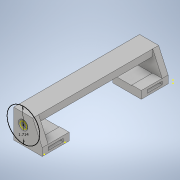
# Autodesk Inventor part: GRAVVY FRONT
Saved by Autodesk Inventor 2020 (Build 240168000, 168)
## iProperties
Created: 2019-11-03
Part Number: GRAVVY FRONT
Material: Generic
Document SubType Name: Modeling
Designer: Arman Ahmad
Density: 1 g/cm^3
Appearance: Default
Author: Arman Ahmad
## iProperties of the stored document _3DPrint.ipt
Created: 2020-02-16
Part Number: _3DPrint
Material: Generic
Document SubType Name: Modeling
Designer: akend
Density: 1 g/cm^3
Appearance: Default
Author: akend
Autodesk Inventor part; units mm, degrees
ref_plane "YZ Plane" through (0, 0, 0) normal (1, 0, 0) x (0, 1, 0)
ref_plane "XZ Plane" through (0, 0, 0) normal (0, 1, 0) x (-1, 0, 0)
ref_plane "XY Plane" through (0, 0, 0) normal (0, 0, 1) x (1, 0, 0)
sketch "Sketch1" plane through (0, 0, 0) normal (0, 1, 0) x (-1, 0, 0)
  line L0 (41.275, -164.3062) -> (9.525, -164.3062)
  line L1 (9.525, -164.3062) -> (9.525, -11.9062)
  line L2 (9.525, -11.9062) -> (41.275, -11.9062)
  line L3 (41.275, -11.9062) -> (41.275, -164.3062)
  line L4 (41.275, -164.3062) -> (9.525, -164.3062)
  line L5 (9.525, -164.3062) -> (9.525, -146.7428)
  line L6 (9.525, -146.7428) -> (41.275, -146.7428)
  line L7 (41.275, -146.7428) -> (41.275, -164.3062)
  point P0 (0, 0)
  dimension "d37" = 31.75
  dimension "d50" = 152.4
  constraints: 16 end point, 4 parallel, 2 horizontal, 2 perpendicular, 1 point on line
  measures "d37" distance between parallel lines of L1 L3
  measures "d50" distance between parallel lines of L0 L2
sketch "Sketch2" plane through (0, 0, 0) normal (1, 0, 0) x (0, 1, 0)
  point P0 (0, 0)
extrude "Extrusion1" add sketch "Sketch1" along normal mid plane 7.62
sketch "Sketch3" plane through (0, 3.81, 0) normal (0, 1, 0) x (1, 0, 0)
  point P0 (0, 0)
sketch "Sketch4" plane through (0, 3.81, 0) normal (0, 1, 0) x (1, 0, 0)
  line L0 (-47.625, 3.9687) -> (-47.625, 172.2437)
  line L1 (-47.625, 172.2437) -> (-3.175, 172.2437)
  line L2 (-3.175, 172.2437) -> (-3.175, 3.9688)
  line L3 (-41.275, 164.3062) -> (-9.525, 164.3062) projected
  line L4 (-41.275, 11.9062) -> (-41.275, 164.3062) projected
  line L5 (-9.525, 164.3062) -> (-41.275, 164.3062) projected
  line L6 (-41.275, 11.9062) -> (-9.525, 11.9062) projected
  line L7 (-41.275, 164.3062) -> (-9.525, 164.3062)
  line L8 (-9.525, 164.3062) -> (-9.525, 11.9062)
  line L9 (-9.525, 11.9062) -> (-41.275, 11.9062)
  line L10 (-41.275, 11.9062) -> (-41.275, 164.3062)
  line L11 (-47.625, 3.9687) -> (-3.175, 3.9688)
  dimension "d38" = 7.9375
  dimension "d40" = 7.9375
  dimension "d41" = 6.35
  dimension "d42" = 6.35
  constraints: 16 end point, 4 parallel, 1 horizontal, 1 perpendicular, 1 vertical
  measures "d38" distance between parallel lines of L3 L1
  measures "d40" distance between parallel lines of L11 L6
  measures "d41" distance between parallel lines of L4 L0
  measures "d42" distance between parallel lines of L8 L2
extrude "Extrusion2" add sketch "Sketch4" against normal blind 38.1
fillet "Fillet1" radius 3.175 3 edges at (-47.625, -34.29, -88.1062) (-47.625, -15.24, -3.9687) (-47.625, -15.24, -172.2437)
sketch "Sketch6" plane through (-3.175, 3.81, -3.9688) normal (1, 0, 0) x (0, 0, -1)
  line L0 (140.3375, -7.0861) -> (160.3375, -7.0861)
  line L1 (160.3375, -7.0861) -> (160.3375, -3.0861)
  line L2 (160.3375, -3.0861) -> (140.3375, -3.0861)
  line L3 (140.3375, -3.0861) -> (140.3375, -7.0861)
  line L4 (27.3343, -7.0861) -> (7.3343, -7.0861)
  line L5 (7.3343, -7.0861) -> (7.3343, -3.0861)
  line L6 (7.3343, -3.0861) -> (27.3343, -3.0861)
  line L7 (27.3343, -3.0861) -> (27.3343, -7.0861)
  line L8 (85.181, -7.0861) -> (65.181, -7.0861)
  line L9 (65.181, -7.0861) -> (65.181, -3.0861)
  line L10 (65.181, -3.0861) -> (85.181, -3.0861)
  line L11 (85.181, -3.0861) -> (85.181, -7.0861)
  line L12 (0, 0) -> (168.275, 0) projected
  point P0 (-3.9688, -3.81)
  point P1 (160.3375, -38.1)
  dimension "d20" = 4
  dimension "d21" = 20
  dimension "d22" = 0
  dimension "d23" = 3.0861
  dimension "d24" = 3.0861
  constraints: 24 end point, 6 parallel, 3 equal length, 3 horizontal, 3 perpendicular, 2 point on line
  measures "d20" distance between parallel lines of L2 L0
  measures "d21" distance between parallel lines of L3 L1
  measures "d22" distance from line of point (160.337, -38.1) L1
  measures "d23" distance between parallel lines of L12 L2
  measures "d24" distance between parallel lines of L12 L10
extrude "Extrusion3" cut sketch "Sketch6" against normal blind 31.75 contours L3 L2 L1 L0
sketch "Sketch7" plane through (-3.175, 3.81, -3.9688) normal (1, 0, 0) x (0, 0, -1)
  line L0 (27.9375, -7.0861) -> (7.9375, -7.0861)
  line L1 (7.9375, -7.0861) -> (7.9375, -3.0861)
  line L2 (7.9375, -3.0861) -> (27.9375, -3.0861)
  line L3 (27.9375, -3.0861) -> (27.9375, -7.0861)
  line L4 (160.3375, -7.0861) -> (140.3375, -7.0861) projected
  line L5 (140.3375, -7.0861) -> (140.3375, -3.0861) projected
  line L6 (0, 0) -> (168.275, 0) projected
  line L7 (140.3375, -3.0861) -> (160.3375, -3.0861) projected
  point P0 (-3.9688, -3.81)
  point P1 (7.9375, -38.1)
  dimension "d28" = 0
  dimension "d31" = 3.0861
  constraints: 8 end point, 3 parallel, 2 equal length, 1 horizontal, 1 perpendicular
  measures "d28" distance from line of L1 point (7.937, -38.1)
  measures "d31" distance between parallel lines of L6 L2
extrude "Extrusion4" cut sketch "Sketch7" against normal blind 31.75
sketch "Sketch8" plane through (-3.175, 3.81, -3.9688) normal (1, 0, 0) x (0, 0, -1)
  line L0 (94.1324, -7.0861) -> (74.1324, -7.0861)
  line L1 (74.1324, -7.0861) -> (74.1324, -3.0861)
  line L2 (74.1324, -3.0861) -> (94.1324, -3.0861)
  line L3 (94.1324, -3.0861) -> (94.1324, -7.0861)
  line L4 (140.3375, -7.0861) -> (140.3375, -3.0861) projected
  line L5 (140.3375, -3.0861) -> (160.3375, -3.0861) projected
  line L6 (0, 0) -> (168.275, 0) projected
  line L7 (168.275, 0) -> (168.275, -38.1) projected
  line L8 (0, 0) -> (0, -38.1) projected
  point P0 (-3.9688, -3.81)
  point P1 (0, -38.1)
  dimension "d32" = 3.0861
  dimension "d33" = 74.1426
  constraints: 8 end point, 4 parallel, 1 horizontal, 1 perpendicular, 1 other
  measures "d32" distance between parallel lines of L6 L2
  measures "d33" distance between parallel lines of L7 L3
extrude "Extrusion5" cut sketch "Sketch8" against normal blind 31.75
sketch "Sketch10" plane through (-3.175, -34.29, -172.2437) normal (0, 0, -1) x (-1, 0, 0)
  point P0 (-3.175, 34.29)
  point P1 (24.9089, 14.3132)
hole "Hole3" at (-28.0839, -19.9768, -172.2437) direction (0, 0, 1) diameter 8.89 end through all
sketch "Sketch11" plane through (-3.175, -34.29, -172.2437) normal (0, 0, -1) x (-1, 0, 0)
  circle A0 centre (24.9089, 14.3132) radius 4.445 projected
  point P0 (-3.175, 34.29)
  constraints: 1 coincident
hole "Hole4" at (-28.0839, -19.9768, -172.2437) direction (0, 0, 1) diameter 12.7 depth 4.7625 tip angle 118
sketch "Sketch12" plane through (-3.175, -34.29, -3.9688) normal (0, 0, 1) x (1, 0, 0)
  point P0 (3.175, 34.29)
  point P1 (-25.0763, 13.995)
hole "Hole5" at (-28.2513, -20.295, -3.9688) direction (0, 0, -1) diameter 12.7 depth 4.7625 tip angle 118
sketch "Sketch13" plane through (-47.625, 3.81, -169.0687) normal (-1, 0, 0) x (0, 0, 1)
  line L0 (74.93, -14.0718) -> (86.995, -14.0718)
  line L1 (86.995, -14.0718) -> (86.995, -8.3898)
  line L2 (86.995, -8.3898) -> (74.93, -8.3898)
  line L3 (74.93, -8.3898) -> (74.93, -14.0718)
  line L4 (161.925, 0) -> (161.925, -34.925) projected
  line L5 (0, -34.925) -> (0, 0) projected
  point P0 (169.0687, -3.81)
  dimension "d72" = 74.93
  dimension "d73" = 74.93
  constraints: 8 end point, 2 parallel, 1 horizontal, 1 perpendicular
  measures "d72" distance between parallel lines of L4 L1
  measures "d73" distance between parallel lines of L5 L3
extrude "Extrusion6" add sketch "Sketch13" along normal blind 12.7
fillet "Fillet2" radius 1.27 1 edges at (-60.325, -10.2618, -88.1062)
fillet "Fillet3" radius 1.27 9 edges at (-60.325, -4.5798, -88.1062) (-59.953, -9.8898, -94.1387) (-60.325, -6.7858, -94.1387) (-53.34, -10.2618, -94.1387) (-53.975, -4.5798, -94.1387) (-59.953, -9.8898, -82.0737) (-60.325, -6.7858, -82.0737) (-53.34, -10.2618, -82.0737) (-53.975, -4.5798, -82.0737)
sketch "Sketch14" plane through (-47.625, -10.2618, -92.8687) normal (0, -1, 0) x (1, 0, 0)
  point P0 (47.625, 92.8687)
  point P1 (-5.4964, 5.0244)
hole "Hole6" at (-53.1214, -10.2618, -87.8444) direction (0, 1, 0) diameter 6.35 end through all
sketch "Sketch15" plane through (0, -34.29, 0) normal (0, -1, 0) x (1, 0, 0)
  line L0 (-3.175, -164.3062) -> (-34.925, -164.3062) projected
  line L1 (-3.175, -172.2437) -> (-3.175, -3.9688) projected
  line L2 (-9.6565, -164.3062) -> (-3.175, -164.3062)
  line L3 (-3.175, -164.3062) -> (-3.175, -12.0649)
  line L4 (-3.175, -12.0649) -> (-9.6565, -12.0649)
  line L5 (-9.6565, -12.0649) -> (-9.6565, -164.3062)
  point P0 (0, 0)
  constraints: 8 end point, 2 parallel, 2 point on line, 1 horizontal, 1 perpendicular
extrude "Extrusion7" cut sketch "Sketch15" against normal blind 21.59
sketch "Sketch16" plane through (0, -34.29, 0) normal (0, -1, 0) x (1, 0, 0)
  line L0 (-41.275, -11.9062) -> (-41.275, -164.3062) projected
  line L1 (-47.625, -169.0687) -> (-47.625, -7.1438) projected
  line L2 (-41.275, -164.3062) -> (-47.625, -164.3062)
  line L3 (-47.625, -164.3062) -> (-47.625, -11.6343)
  line L4 (-47.625, -11.6343) -> (-41.275, -11.6343)
  line L5 (-41.275, -11.6343) -> (-41.275, -164.3062)
  point P0 (0, 0)
  constraints: 8 end point, 2 parallel, 1 horizontal, 1 perpendicular, 1 point on line
extrude "Extrusion8" cut sketch "Sketch16" against normal blind 21.59
fillet "Fillet4" radius 1.27 4 edges at (-3.175, -34.29, -8.0168) (-3.175, -15.24, -3.9688) (-3.175, -34.29, -168.275) (-3.175, -15.24, -172.2437)
sketch "Sketch17" plane through (-44.45, -34.29, -3.9687) normal (0, 0, 1) x (1, 0, 0)
  line L0 (3.6661, -9.4735) -> (29.0661, -9.4735)
  line L1 (29.0661, -9.4735) -> (29.0661, 38.1)
  line L2 (29.0661, 38.1) -> (3.6661, 38.1)
  line L3 (3.6661, 38.1) -> (3.6661, -9.4735)
  circle A0 centre (16.3661, 14.3132) radius 4.445 projected
  line L4 (3.6661, -9.4735) -> (29.0661, 38.1) construction
  line L5 (29.0661, -9.4735) -> (3.6661, 38.1) construction
  line L6 (3.6661, 38.1) -> (-19.5186, 38.1)
  line L7 (-19.5186, 38.1) -> (-19.5186, -9.4735)
  line L8 (-19.5186, -9.4735) -> (3.6661, -9.4735)
  line L9 (3.6661, -9.4735) -> (3.6661, 38.1)
  line L10 (29.0661, 38.1) -> (55.1329, 38.1)
  line L11 (55.1329, 38.1) -> (55.1329, -9.4735)
  line L12 (55.1329, -9.4735) -> (29.0661, -9.4735)
  line L13 (29.0661, -9.4735) -> (29.0661, 38.1)
  point P0 (44.45, 34.29)
  point P1 (29.0661, -9.4735)
  point P2 (3.6661, -9.4735)
  dimension "d90" = 25.4
  constraints: 28 end point, 6 parallel, 3 horizontal, 3 perpendicular, 2 midpoint, 1 point on line
  measures "d90" distance of L0.start L0.end
extrude "Extrusion9" cut sketch "Sketch17" against normal blind 169.8625 contours L8 L7 L6 L3 | L1 L10 L11 L12
sketch "Sketch18" plane through (-15.3839, 3.81, -172.2437) normal (0, 0, -1) x (-1, 0, 0)
  circle A0 centre (12.7, -23.7868) radius 4.445 projected
  circle A1 centre (12.7, -23.7868) radius 21.7714
  point P0 (-15.3839, -3.81)
  dimension "d93" = 43.5429
  constraints: 1 centre point, 1 coincident
  measures "d93" diameter of A1
sketch "Sketch19" plane through (-34.925, -3.2761, -144.3062) normal (0, 0, -1) x (-1, 0, 0)
  point P0 (-34.925, 3.2761)
sketch "Sketch20" plane through (0, -3.81, 0) normal (0, -1, 0) x (1, 0, 0)
  line L0 (-40.7839, -164.3062) -> (-15.3839, -164.3062) projected
  line L1 (-40.7839, -11.9062) -> (-15.3839, -11.9062) projected
  line L2 (-40.7839, -164.3062) -> (-15.3839, -164.3062)
  line L3 (-15.3839, -164.3062) -> (-15.3839, -11.9062)
  line L4 (-15.3839, -11.9062) -> (-40.7839, -11.9062)
  line L5 (-40.7839, -11.9062) -> (-40.7839, -164.3062)
  point P0 (0, 0)
  constraints: 8 end point, 2 parallel, 1 horizontal, 1 perpendicular
extrude "Extrusion10" add sketch "Sketch20" along normal blind 3
sketch "Sketch21" plane through (0, -6.81, 0) normal (0, -1, 0) x (1, 0, 0)
  line L0 (-40.7839, -164.3062) -> (-40.7839, -172.2437) projected
  line L1 (-40.7839, -164.3062) -> (-34.4339, -164.3062)
  line L2 (-34.4339, -164.3062) -> (-34.4339, -11.9062)
  line L3 (-34.4339, -11.9062) -> (-40.7839, -11.9062)
  line L4 (-40.7839, -11.9062) -> (-40.7839, -164.3062)
  line L5 (-15.3839, -164.3062) -> (-21.7339, -164.3062)
  line L6 (-21.7339, -164.3062) -> (-21.7339, -11.9062)
  line L7 (-21.7339, -11.9062) -> (-15.3839, -11.9062)
  line L8 (-15.3839, -11.9062) -> (-15.3839, -164.3062)
  point P0 (0, 0)
  dimension "d96" = 6.35
  dimension "d97" = 6.35
  constraints: 16 end point, 4 parallel, 2 horizontal, 2 perpendicular, 1 point on line
  measures "d96" distance of L3.end L2.end
  measures "d97" distance of L6.end L7.end
extrude "Extrusion11" add sketch "Sketch21" along normal blind 8.255
sketch "Sketch22" plane through (-15.3839, -34.29, -3.9688) normal (1, 0, 0) x (0, 0, -1)
  point P0 (-3.9688, 34.29)
sketch "Sketch23" plane through (-15.3839, -34.29, -3.9688) normal (1, 0, 0) x (0, 0, -1)
  line L0 (168.275, 38.1) -> (0, 38.1) projected
  line L1 (0, 38.1) -> (35.8902, 38.1)
  line L2 (35.8902, 38.1) -> (35.8902, 27.9146)
  line L3 (35.8902, 27.9146) -> (0, 27.9146)
  line L4 (0, 27.9146) -> (0, 38.1)
  line L5 (168.275, 38.1) -> (132.3848, 38.1)
  line L6 (132.3848, 38.1) -> (132.3848, 27.9146)
  line L7 (132.3848, 27.9146) -> (168.275, 27.9146)
  line L8 (168.275, 27.9146) -> (168.275, 38.1)
  line L9 (7.9375, 35.0139) -> (7.9375, 31.0139) projected
  line L10 (7.9375, 31.0139) -> (27.9375, 31.0139) projected
  line L11 (7.9375, 35.0139) -> (27.9375, 35.0139)
  line L12 (27.9375, 35.0139) -> (27.9375, 31.0139)
  line L13 (27.9375, 31.0139) -> (7.9375, 31.0139)
  line L14 (7.9375, 31.0139) -> (7.9375, 35.0139)
  line L15 (160.3375, 35.0139) -> (140.3375, 35.0139) projected
  line L16 (140.3375, 31.0139) -> (160.3375, 31.0139) projected
  line L17 (140.3375, 35.0139) -> (160.3375, 35.0139)
  line L18 (160.3375, 35.0139) -> (160.3375, 31.0139)
  line L19 (160.3375, 31.0139) -> (140.3375, 31.0139)
  line L20 (140.3375, 31.0139) -> (140.3375, 35.0139)
  point P0 (-3.9688, 34.29)
  dimension "d100" = 35.8902
  dimension "d101" = 10.1854
  dimension "d102" = 35.8902
  dimension "d103" = 10.1854
  constraints: 32 end point, 8 parallel, 4 horizontal, 4 perpendicular
  measures "d100" distance of L2.end L3.end
  measures "d101" distance of L1.end L2.end
  measures "d102" distance of L7.end L6.end
  measures "d103" distance of L6.end L5.end
extrude "Extrusion12" add sketch "Sketch23" along normal blind 12.7
sketch "Sketch24" plane through (0, -34.29, 0) normal (0, -1, 0) x (1, 0, 0)
  line L0 (-15.3839, -164.3062) -> (-21.7339, -164.3062) projected
  line L1 (-40.7839, -172.2437) -> (-40.7839, -3.9687) projected
  line L2 (-15.3839, -164.3062) -> (-40.7839, -164.3062)
  line L3 (-40.7839, -164.3062) -> (-40.7839, -11.9062)
  line L4 (-40.7839, -11.9062) -> (-15.3839, -11.9062)
  line L5 (-15.3839, -11.9062) -> (-15.3839, -164.3062)
  point P0 (0, 0)
  constraints: 8 end point, 2 parallel, 1 horizontal, 1 perpendicular, 1 point on line
extrude "Extrusion13" cut sketch "Sketch24" against normal blind 28.575
sketch "Sketch25" plane through (-40.7839, -34.29, -164.3062) normal (0, 0, 1) x (1, 0, 0)
  line L0 (25.4, 0) -> (25.4, 27.9146) projected
  line L1 (0, 0) -> (0, 38.1) projected
  line L2 (25.4, 0) -> (0, 0)
  line L3 (0, 0) -> (0, 3.175)
  line L4 (0, 3.175) -> (25.4, 3.175)
  line L5 (25.4, 3.175) -> (25.4, 0)
  line L6 (25.4, 0) -> (21.59, 0)
  line L7 (21.59, 0) -> (21.59, 8.89)
  line L8 (21.59, 8.89) -> (25.4, 8.89)
  line L9 (25.4, 8.89) -> (25.4, 0)
  line L10 (0, 0) -> (3.81, 0)
  line L11 (3.81, 0) -> (3.81, 8.89)
  line L12 (3.81, 8.89) -> (0, 8.89)
  line L13 (0, 8.89) -> (0, 0)
  point P0 (40.7839, 34.29)
  point P1 (25.4, 8.89)
  point P2 (21.59, 3.175)
  point P3 (3.81, 3.175)
  point P4 (0, 8.89)
  dimension "d108" = 3.175
  dimension "d109" = 3.81
  dimension "d110" = 8.89
  dimension "d111" = 3.81
  dimension "d112" = 8.89
  constraints: 24 end point, 6 parallel, 3 horizontal, 3 perpendicular, 1 point on line
  measures "d108" distance of L2.end L3.end
  measures "d109" distance of L7.end L8.end
  measures "d110" distance of L6.end L7.end
  measures "d111" distance of L12.end L11.end
  measures "d112" distance of L11.end L10.end
extrude "Extrusion14" add sketch "Sketch25" along normal blind 152.4
sketch "Sketch26" plane through (0, 3.81, 0) normal (0, 1, 0) x (1, 0, 0)
  line L0 (-2.6839, 3.9687) -> (-2.6839, 39.8589) projected
  line L1 (-40.7839, 164.3062) -> (-40.7839, 11.9062) projected
  line L2 (-2.6839, 39.8589) -> (-40.7839, 39.8589)
  line L3 (-40.7839, 39.8589) -> (-40.7839, 136.3535)
  line L4 (-40.7839, 136.3535) -> (-2.6839, 136.3535)
  line L5 (-2.6839, 136.3535) -> (-2.6839, 39.8589)
  point P0 (0, 0)
  dimension "d115" = 96.4946
  constraints: 8 end point, 2 parallel, 1 horizontal, 1 perpendicular, 1 point on line
  measures "d115" distance of L2.end L3.end
extrude "Extrusion15" cut sketch "Sketch26" against normal blind 11.1125
sketch "Sketch27" plane through (-40.7839, -34.29, -3.9687) normal (-1, 0, 0) x (0, 0, 1)
  point P0 (3.9688, 34.29)
sketch "Sketch28" plane through (-40.7839, -34.29, -3.9687) normal (0, 0, 1) x (1, 0, 0)
  line L0 (25.4, 27.9146) -> (38.1, 27.9146) projected
  line L1 (25.4, 27.9146) -> (25.4, 0) projected
  line L2 (38.1, 27.9146) -> (25.4, 0)
  line L3 (25.4, 27.9146) -> (25.4, 28.575) projected
  line L4 (25.4, 0) -> (25.4, 27.9146)
  line L5 (38.1, 38.1) -> (38.1, 27.9146) projected
  line L6 (25.4, 27.9146) -> (38.1, 27.9146)
  point P0 (40.7839, 34.29)
  constraints: 6 end point, 1 collinear, 1 perpendicular
extrude "Extrusion16" add sketch "Sketch28" against normal blind 7.9375
sketch "Sketch29" plane through (-40.7839, -5.715, -164.3062) normal (0, 0, 1) x (1, 0, 0)
  line L0 (25.4, -28.575) -> (0, -28.575) projected
  line L1 (25.4, -0.6604) -> (25.4, -28.575) projected
  line L2 (25.4, -28.575) -> (25.4, -0.6604)
  line L3 (38.1, -0.6604) -> (25.4, -0.6604) projected
  line L4 (25.4, -0.6604) -> (38.1, -0.6604)
  line L5 (38.1, -0.6604) -> (25.4, -28.575) projected
  line L6 (38.1, -0.6604) -> (25.4, -28.575)
  point P0 (40.7839, 5.715)
  constraints: 6 end point, 2 collinear, 1 vertical
extrude "Extrusion17" add sketch "Sketch29" against normal blind 7.9375
sketch "Sketch30" plane through (-40.7839, -25.4, -164.3062) normal (0, 1, 0) x (1, 0, 0)
  line L0 (3.81, 0) -> (3.81, -152.4) projected
  line L1 (25.4, 0) -> (0, 0) projected
  line L2 (3.81, -152.4) -> (6.35, -152.4)
  line L3 (6.35, -152.4) -> (6.35, 0)
  line L4 (6.35, 0) -> (3.81, 0)
  line L5 (3.81, 0) -> (3.81, -152.4)
  line L6 (21.59, 0) -> (21.59, -152.4) projected
  line L7 (21.59, -152.4) -> (19.05, -152.4)
  line L8 (19.05, -152.4) -> (19.05, 0)
  line L9 (19.05, 0) -> (21.59, 0)
  line L10 (21.59, 0) -> (21.59, -152.4)
  point P0 (40.7839, -164.3062)
  dimension "d122" = 2.54
  dimension "d123" = 2.54
  constraints: 16 end point, 4 parallel, 2 horizontal, 2 perpendicular, 2 point on line
  measures "d122" distance of L4.end L3.end
  measures "d123" distance of L8.end L9.end
extrude "Extrusion18" add sketch "Sketch30" against normal blind 7.9375
fillet "Fillet5" radius 2.54 2 edges at (-34.4339, -25.4, -88.1062) (-21.7339, -25.4, -88.1062)
sketch "Sketch31" plane through (-40.7839, -25.4, -11.9062) normal (0, 1, 0) x (1, 0, 0)
  circle A0 centre (-3.2262, 76.2) radius 2.921
  line L0 (-6.4525, 80.645) -> (-6.4525, 71.755)
  line L1 (-6.4525, 71.755) -> (0, 71.755)
  line L2 (0, 71.755) -> (0, 80.645)
  line L3 (0, 80.645) -> (-6.4525, 80.645)
  line L4 (-6.4525, 80.645) -> (0, 71.755) construction
  line L5 (-6.4525, 71.755) -> (0, 80.645) construction
  point P0 (40.7839, -11.9062)
  dimension "d127" = 5.842
  dimension "d128" = 8.89
  constraints: 12 end point, 2 midpoint, 2 parallel, 1 centre point, 1 perpendicular, 1 vertical
  measures "d127" diameter of A0
  measures "d128" distance of L0.start L0.end
extrude "Extrusion19" add sketch "Sketch31" against normal blind 4.7625
sketch "Sketch32" plane through (-40.7839, -34.29, -172.2437) normal (0, 0, -1) x (-1, 0, 0)
  point P0 (-40.7839, 34.29)
sketch "Sketch33" plane through (0, -34.29, 0) normal (0, -1, 0) x (1, 0, 0)
  line L0 (-40.7839, -3.9687) -> (-40.7839, -172.2437) projected
  line L1 (-55.97, -106.4068) -> (-40.7839, -106.4068)
  line L2 (-40.7839, -106.4068) -> (-40.7839, -77.2514)
  line L3 (-40.7839, -77.2514) -> (-55.97, -77.2514)
  line L4 (-55.97, -77.2514) -> (-55.97, -106.4068)
  point P0 (0, 0)
  constraints: 8 end point, 2 parallel, 1 horizontal, 1 perpendicular, 1 point on line
extrude "Extrusion20" cut sketch "Sketch33" against normal blind 25.4
body "Solid1"
